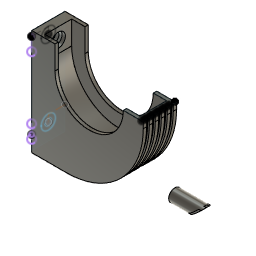
HQ7-Holder v1 (Autodesk Fusion 360 design; units mm, degrees)
Autodesk Fusion 360 part; units mm, degrees
note: some values were not read from the file. Chosen so that the rebuilt part matches the saved one: which bodies a step acts on.
sketch "circle" plane through (0, 0, 0) normal (0, 1, 0) x (1, 0, 0)
  circle A0 centre (0, -40) radius 27.5
  dimension "d1" = 55
  measures "d1" diameter of A0
sketch "Sketch2" plane through (0, 0, 0) normal (0, 1, 0) x (1, 0, 0)
  line L0 (0, -40) -> (-20.5, -40) construction
  arc A0 (28.5, -40) -> (-28.5, -40) centre (0, -40) ccw
  line L1 (0, -11.5) -> (0, -5.5)
  line L2 (0, -5.5) -> (0, 2.5)
  line L3 (-34.5, 8.5) -> (-34.5, -40)
  line L4 (28.5, -40) -> (31.5, -40)
  line L5 (31.5, -40) -> (31.5, -36.5)
  line L6 (-13.5, 8.5) -> (-34.5, 8.5)
  arc A1 (31.5, -36.5) -> (-13.5, 8.5) centre (-13.5, -36.5) ccw
  line L7 (28.5, -40) -> (20.5, -40)
  arc A2 (20.5, -40) -> (-20.5, -40) centre (0, -40) ccw
  line L8 (-34.5, -40) -> (-34.5, -43)
  line L9 (-34.5, -43) -> (-34.5, -51)
  line L10 (-34.5, -51) -> (-34.5, -54)
  line L11 (-34.5, -54) -> (-20.5, -54)
  line L12 (-20.5, -54) -> (-20.5, -40)
  line L13 (-28.5, -40) -> (-28.5, -54)
  point P0 (0, -40)
  dimension "d14" = 28.5
  dimension "d15" = 6
  dimension "d16" = 6
  dimension "d17" = 8
  dimension "d19" = 3
  dimension "d20" = 45
  dimension "d21" = 8
  dimension "d22" = 3
  dimension "d23" = 8
  dimension "d24" = 3
  constraint coincident P0 L0.start
  constraint horizontal L0
  constraint midpoint A0 L1.start
  constraint vertical L1
  constraint vertical L2
  constraint perpendicular L3 L6
  constraint tangent L5 A1
  constraint tangent L6 A1
  constraint parallel L4 L7
  constraint parallel L8 L9
  constraint parallel L9 L10
  constraint perpendicular L10 L11
  constraint tangent A2 L12
  constraint coincident L11 L13.end
  constraint tangent A0 L13
  measures "d14" distance of P0 A0.end
  measures "d15" distance of A0.end L3.end
  measures "d16" distance of L1.start L1.end
  measures "d17" distance of L1.end L2.end
  measures "d19" distance of A0.start L4.end
  measures "d20" radius of A1
  measures "d21" distance of A0.start L7.end
  measures "d22" distance of L3.end L8.end
  measures "d23" distance of L8.end L9.end
  measures "d24" distance of L9.end L10.end
extrude "Extrude2" add sketch "Sketch2" along normal blind 20 contours A0 L3 L4 L5 L6 A1 L8 L9 L10 L11 L13 makes body 1
extrude "Extrude3" add sketch "Sketch2" along normal blind 2 contours A0 L7 A2 L11 L12 L13 bodies 1
extrude "Extrude4" add sketch "Sketch2" against normal blind 2 from surface at 20 contours A0 L7 A2 L11 L12 L13 bodies 1
sketch "Sketch3" plane through (-34.5, 0, 0) normal (-1, 0, 0) x (0, -1, 0)
  line L0 (0, -8.5) -> (0, 54)
  line L1 (0, 54) -> (-20, 54)
  line L2 (-20, 54) -> (-20, -8.5)
  line L3 (-20, -8.5) -> (0, -8.5)
  line L4 (0, 5.5) -> (0, -2.5)
  line L5 (-20, 5.5) -> (-10, 5.5) construction
  line L6 (-10, 5.5) -> (-10, 1.5) construction
  circle A0 centre (-10, 1.5) radius 4.25
  line L7 (0, 43) -> (0, 51)
  line L8 (0, 51) -> (-10, 51) construction
  line L9 (-10, 51) -> (-10, 47) construction
  circle A1 centre (-10, 47) radius 4.25
  circle A2 centre (-10, 47) radius 1.9
  circle A3 centre (-10, 1.5) radius 1.9
  dimension "d32" = 10
  dimension "d33" = 4
  dimension "d34" = 8.5
  dimension "d35" = 10
  dimension "d36" = 4
  dimension "d37" = 8.5
  dimension "d40" = 3.8
  dimension "d41" = 3.8
  constraint coincident L2 L5.start
  constraint perpendicular L2 L5
  constraint coincident L6.end A0.centre
  constraint coincident L7.end L8.start
  constraint perpendicular L7 L8
  constraint perpendicular L8 L9
  constraint coincident L9.end A1.centre
  constraint concentric A1 A2
  constraint concentric A0 A3
  measures "d32" distance of L5.start L5.end
  measures "d33" distance of L5.end L6.end
  measures "d34" diameter of A0
  measures "d35" distance of L7.end L8.end
  measures "d36" distance of L8.end L9.end
  measures "d37" diameter of A1
  measures "d40" diameter of A2
  measures "d41" diameter of A3
extrude "Extrude6" cut sketch "Sketch3" against normal blind 70 contours A2 | A3 bodies 1
extrude "Extrude5" cut sketch "Sketch3" against normal blind 15 contours A1 | A2 bodies 1
extrude "Extrude7" add sketch "Sketch3" against normal blind 4 contours A1 bodies 1
chamfer "Chamfer1" distance 2 distance2 1.8 1 edges at (-30.5, 11.7714, 46.3129) measured on face at (-30.5, 6.5562, 46.6945) on bodies 1
fillet "Fillet1" radius 4 1 edges at (-30.5, 13.6361, 48.4103) on bodies 1
extrude "Extrude8" cut sketch "Sketch3" against normal blind 64 from surface at -10 contours A0 bodies 1
extrude "Extrude9" add sketch "Sketch3" against normal blind 21 from surface at -35 separate body contours A0 | A3 makes body 2
split "Split1" by face at (2.3845, 9.9767, -5.6032) of body 1 bodies 2 makes body 3 at (17.3828, 5.7811, 2.0133)
move_body "Move1" bodies 2 to x (1, 0, 0) y (0, 1, 0) z (0, 0, 1) at (0, 0, 0)
chamfer "Chamfer2" distance 2 distance2 2 1 edges at (-24.5, 11.7714, 2.1871) measured on face at (-31.1667, 8.1094, 1.3108) on bodies 1
fillet "Fillet2" radius 5 1 edges at (-24.5, 13.6361, 2.9103) on bodies 1
move_body "Move2" bodies 2 to x (1, 0, 0) y (0, 1, 0) z (0, 0, 1) at (-97, 0, 0)
move_body "Move3" bodies 2 to x (1, 0, 0) y (0, 1, 0) z (0, 0, 1) at (97, 0, 0)
sketch "Sketch4" plane through (0, 0, 40) normal (0, 0, 1) x (-1, 0, 0)
  line L0 (-20.5, 0) -> (-31.5, 0)
  line L1 (-31.5, 0) -> (-31.5, -20)
  line L2 (-31.5, -20) -> (-20.5, -20)
  line L3 (-20.5, -20) -> (-20.5, -18)
  line L4 (-20.5, -18) -> (-28.5, -18)
  line L5 (-28.5, -18) -> (-28.5, -2)
  line L6 (-28.5, -2) -> (-20.5, -2)
  line L7 (-20.5, -2) -> (-20.5, 0)
  line L8 (-31.5, -20) -> (-32.5, -20)
  line L9 (-32.5, -20) -> (-32.5, -18)
  line L10 (-32.5, -18) -> (-31.5, -18)
  line L11 (-31.5, -18) -> (-31.5, -20)
  line L12 (-31.5, -16.4) -> (-32.5, -16.4)
  line L13 (-32.5, -16.4) -> (-32.5, -14.4)
  line L14 (-32.5, -14.4) -> (-31.5, -14.4)
  line L15 (-31.5, -12.8) -> (-32.5, -12.8)
  line L16 (-32.5, -12.8) -> (-32.5, -10.8)
  line L17 (-32.5, -10.8) -> (-31.5, -10.8)
  line L18 (-31.5, -9.2) -> (-32.5, -9.2)
  line L19 (-32.5, -9.2) -> (-32.5, -7.2)
  line L20 (-32.5, -7.2) -> (-31.5, -7.2)
  line L21 (-31.5, -5.6) -> (-32.5, -5.6)
  line L22 (-32.5, -5.6) -> (-32.5, -3.6)
  line L23 (-32.5, -3.6) -> (-31.5, -3.6)
  line L24 (-31.5, -2) -> (-32.5, -2)
  line L25 (-32.5, -2) -> (-32.5, 0)
  line L26 (-32.5, 0) -> (-31.5, 0)
  point P0 (-31.5, -16.4)
  point P1 (-31.5, -12.8)
  point P2 (-31.5, -9.2)
  point P3 (-31.5, -5.6)
  point P4 (-31.5, -2)
  dimension "d60" = 1
  dimension "d61" = 2
  dimension "d64" = 0
  dimension "d65" = 18
  constraint horizontal L8
  constraint vertical L9
  constraint horizontal L10
  constraint vertical L11
  constraint coincident L1.end L2.start
  measures "d60" distance of L1.end L8.end
  measures "d61" distance of L1.end L10.end
sketch "Sketch5" plane through (0, 0, 0) normal (0, -1, 0) x (1, 0, 0)
  line L0 (31.5, 40) -> (20.5, 40)
  arc A0 (-20.5, 40) -> (20.5, 40) centre (0, 40) ccw
  line L1 (-20.5, 40) -> (-20.5, 54)
  line L2 (-20.5, 54) -> (-34.5, 54)
  line L3 (-34.5, 54) -> (-34.5, -8.5)
  line L4 (-34.5, -8.5) -> (-13.5, -8.5)
  arc A1 (-13.5, -8.5) -> (31.5, 36.5) centre (-13.5, 36.5) ccw
  line L5 (31.5, 36.5) -> (31.5, 40)
sweep "Sweep1" [no effect]
combine "Combine1" operation add target body 1 tool bodies 2 keep tools result as body 4 in component "Component"
sweep "Sweep1'" add profiles "Sketch4" along 3 edges at (31.5, 0, 38.25) (18.3198, 0, 4.6802) (-24, 0, -8.5) section 1 contours L1 L24 L25 L26 | L1 L21 L22 L23 | L1 L18 L19 L20 | L1 L8 L9 L10 L11 | L1 L15 L16 L17 | L1 L12 L13 L14 on bodies 4 bodies 4 in component "Component"
sketch "Sketch6" plane through (0, 0, 0) normal (1, 0, 0) x (0, 1, 0)
  circle A0 centre (10, 1.5) radius 4.25
  point P0 (10, 1.5)
  dimension "d78" = 8.5
  constraint coincident P0 A0.centre
  measures "d78" diameter of A0
extrude "Extrude1" cut sketch "Sketch6" along normal blind 112 thin wall 0.5 inside bodies 4 makes body 5 at (-20.2605, 0, 1.6575) in component "Component"
move_body "Move1'" bodies 4 to x (1, 0, 0) y (0, 1, 0) z (0, 0, 1) at (41, 0, 0) in component "Component"
component "Component" placed x (1, 0, 0) y (0, 1, 0) z (0, 0, 1) at (0, 0, 0)
hidden bodies 1 2 3
equation "d14 = ( 57 / 2 ) * 1 mm"
named bodies: "holder", "SCREW-CAP", "PIPE-HOLDER"
